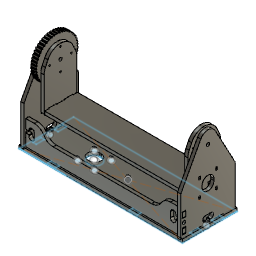
shotbot3 (Autodesk Fusion 360 design; units mm, degrees)
Autodesk Fusion 360 part; units mm, degrees
sketch "basetray sketch" plane through (0, 0, 0) normal (0, 0, 1) x (1, 0, 0) in component "Base Tray"
  line L0 (-147, -27.5) -> (-141, -27.5)
  line L1 (-85.5, -47) -> (-85.5, -41)
  arc A0 (-60.01, -11) -> (-60.01, 11) centre (-60.01, 0) ccw
  line L2 (-60.01, 11) -> (-63.01, 11)
  line L3 (-141, -27.5) -> (-141, -12.5)
  line L4 (-44.51, -14) -> (-47.51, -14)
  line L5 (147, 12.5) -> (147, 27.5)
  line L6 (-85.5, -41) -> (-100.5, -41)
  arc A1 (-78.51, -14) -> (-78.51, -17) centre (-78.51, -15.5) ccw
  line L7 (-100.5, -47) -> (-85.5, -47)
  line L8 (-100.5, -41) -> (-100.5, -47)
  line L9 (-147, 12.5) -> (-141, 12.5)
  line L10 (141, 27.5) -> (141, 12.5)
  arc A2 (-63.01, 11) -> (-63.01, -11) centre (-63.01, 0) ccw
  line L11 (-78.51, -17) -> (-75.51, -17)
  line L12 (-78.51, 14) -> (-75.51, 14)
  arc A3 (-47.51, -14) -> (-47.51, -17) centre (-47.51, -15.5) ccw
  line L13 (-150, 50) -> (150, 50)
  line L14 (-75.51, -14) -> (-78.51, -14)
  line L15 (49.5, -47) -> (64.5, -47)
  line L16 (150, 50) -> (150, -50)
  line L17 (141, 12.5) -> (147, 12.5)
  line L18 (147, -12.5) -> (141, -12.5)
  line L19 (64.5, -41) -> (49.5, -41)
  line L20 (-141, 27.5) -> (-147, 27.5)
  line L21 (-141, -12.5) -> (-147, -12.5)
  circle A4 centre (-144, 0) radius 3
  line L22 (-47.51, -17) -> (-44.51, -17)
  arc A5 (-44.51, -17) -> (-44.51, -14) centre (-44.51, -15.5) ccw
  line L23 (49.5, -41) -> (49.5, -47)
  arc A6 (-75.51, -17) -> (-75.51, -14) centre (-75.51, -15.5) ccw
  line L24 (-75.51, 17) -> (-78.51, 17)
  line L25 (-150, 50) -> (150, -50) construction
  line L26 (64.5, -47) -> (64.5, -41)
  arc A7 (-75.51, 14) -> (-75.51, 17) centre (-75.51, 15.5) ccw
  line L27 (-63.01, -11) -> (-60.01, -11)
  line L28 (-147, 27.5) -> (-147, 12.5)
  line L29 (141, -12.5) -> (141, -27.5)
  circle A8 centre (144, 0) radius 3
  arc A9 (-44.51, 14) -> (-44.51, 17) centre (-44.51, 15.5) ccw
  arc A10 (-47.51, 17) -> (-47.51, 14) centre (-47.51, 15.5) ccw
  line L30 (150, 50) -> (-150, -50) construction
  line L31 (150, -50) -> (-150, -50)
  line L32 (-147, -12.5) -> (-147, -27.5)
  arc A11 (-78.51, 17) -> (-78.51, 14) centre (-78.51, 15.5) ccw
  line L33 (141, -27.5) -> (147, -27.5)
  line L34 (147, -27.5) -> (147, -12.5)
  line L35 (-141, 12.5) -> (-141, 27.5)
  line L36 (-44.51, 17) -> (-47.51, 17)
  line L37 (-47.51, 14) -> (-44.51, 14)
  line L38 (147, 27.5) -> (141, 27.5)
  circle A12 centre (0, 0) radius 2.95
  line L39 (-150, -50) -> (-150, 50)
  constraint horizontal L13
  constraint perpendicular L13 L16
  constraint parallel L13 L31
  constraint parallel L16 L39
  constraint coincident A12.centre L25
  constraint coincident A12.centre L30
  constraint coincident A12.centre origin
sketch "Sketch1" plane through (0, 0, 0) normal (1, 0, 0) x (0, 1, 0) in component "Flange 2"
  line L0 (11, 69.99, -147) -> (11, 66.99, -147)
  arc A0 through (-5, 9, -147) (-10, 14, -147) (-5, 19, -147)
  line L1 (14, 51.49, -147) -> (14, 54.49, -147)
  line L2 (-47, 35.5, -147) -> (-47, 45.5, -147)
  arc A1 through (-17, 54.49, -147) (-15.5, 55.99, -147) (-14, 54.49, -147)
  line L3 (-3.2, 9, -147) -> (-5, 9, -147)
  line L4 (-47, 20.5, -147) -> (-41, 20.5, -147)
  arc A2 through (17, 82.49, -147) (15.5, 80.99, -147) (14, 82.49, -147)
  arc A3 through (5, 19, -147) (10, 14, -147) (5, 9, -147)
  arc A4 through (-17, 85.49, -147) (-15.5, 86.99, -147) (-14, 85.49, -147)
  line L5 (-47, 45.5, -147) -> (-41, 45.5, -147)
  arc A5 through (14, 85.49, -147) (15.5, 86.99, -147) (17, 85.49, -147)
  line L6 (-17, 82.49, -147) -> (-17, 85.49, -147)
  line L7 (17, 85.49, -147) -> (17, 82.49, -147)
  line L8 (-5, 19, -147) -> (5, 19, -147)
  circle A6 through (-2.9, 130, -147) (1.45, 132.5115, -147) (1.45, 127.4885, -147)
  line L9 (12.4, 3, -147) -> (3.2, 3, -147)
  line L10 (5, 9, -147) -> (3.2, 9, -147)
  line L11 (-3.2, 3, -147) -> (-3.2, 9, -147)
  line L12 (-27.3905, -3, -147) -> (-27.6, 3, -147)
  line L13 (-12.6095, -3, -147) -> (-27.3905, -3, -147)
  arc A7 through (14, 54.49, -147) (15.5, 55.99, -147) (17, 54.49, -147)
  line L14 (14, 82.49, -147) -> (14, 85.49, -147)
  arc A8 through (-11, 69.99, -147) (0, 80.99, -147) (11, 69.99, -147)
  line L15 (-41, 35.5, -147) -> (-47, 35.5, -147)
  line L16 (-41, 20.5, -147) -> (-41, 10.5, -147)
  line L17 (-12.4, 3, -147) -> (-12.6095, -3, -147)
  arc A9 through (17, 51.49, -147) (15.5, 49.99, -147) (14, 51.49, -147)
  circle A10 through (-47, 28, -147) (-42.5, 30.5981, -147) (-42.5, 25.4019, -147)
  line L18 (-17, 51.49, -147) -> (-17, 54.49, -147)
  line L19 (27.6, 3, -147) -> (27.3905, -3, -147)
  line L20 (-11, 66.99, -147) -> (-11, 69.99, -147)
  line L21 (-14, 85.49, -147) -> (-14, 82.49, -147)
  arc A11 through (-14, 51.49, -147) (-15.5, 49.99, -147) (-17, 51.49, -147)
  line L22 (27.3905, -3, -147) -> (12.6095, -3, -147)
  arc A12 through (-14, 82.49, -147) (-15.5, 80.99, -147) (-17, 82.49, -147)
  line L23 (-3.2, 3, -147) -> (-12.4, 3, -147)
  line L24 (-41, 45.5, -147) -> (-41, 35.5, -147)
  line L25 (-27.6, 3, -147) -> (-50, 3, -147)
  line L26 (-41, 10.5, -147) -> (-47, 10.5, -147)
  line L27 (12.6095, -3, -147) -> (12.4, 3, -147)
  line L28 (50, 76.6902, -147) -> (50, 3, -147)
  line L29 (-50, 3, -147) -> (-50, 76.6902, -147)
  line L30 (17, 54.49, -147) -> (17, 51.49, -147)
  line L31 (50, 3, -147) -> (27.6, 3, -147)
  line L32 (3.2, 9, -147) -> (3.2, 3, -147)
  arc A13 through (11, 66.99, -147) (0, 55.99, -147) (-11, 66.99, -147)
  line L33 (-47, 10.5, -147) -> (-47, 20.5, -147)
  line L34 (-14, 54.49, -147) -> (-14, 51.49, -147)
  line L35 (50, 76.6902, -147) -> (13.2596, 145.255, -147)
  line L36 (-13.2003, 145.2233, -147) -> (-50, 76.1506, -147)
  arc A14 through (13.2596, 145.255, -147) (0.0202, 153.1703, -147) (-13.2003, 145.2233, -147)
  dimension "d2" = 15
extrude "Extrude1" add sketch "Sketch1" along normal blind 6 contours A0 L3 A3 L8 L9 L10 L11 L12 L13 L17 L19 L22 L23 L25 L27 L28 L29 L31 L32 L35 L36 A14 in plane through (-147, 0, 0) normal (1, 0, 0) makes body 1 in component "Flange 2"
extrude "Extrude1'" add sketch "basetray sketch" along normal blind 6 separate body makes body 2 in component "Base Tray"
sketch "Sketch1 (2)" plane through (0, 0, 0) normal (0, 1, 0) x (1, 0, 0) in component "Back support"
  line L0 (-147, -20.1905, -49) -> (-141, -20.4, -49)
  line L1 (147, -45.1905, -49) -> (147, -35.9095, -49)
  arc A0 through (-125, -25.8, -49) (-130, -20.8, -49) (-135, -25.8, -49)
  line L2 (-135, -27.8, -49) -> (-135, -25.8, -49)
  line L3 (135, -25.8, -49) -> (135, -27.8, -49)
  line L4 (49.5, -5.8, -49) -> (-85.5, -5.8, -49)
  line L5 (49.7095, 0.2, -49) -> (49.5, -5.8, -49)
  arc A1 through (125, -35.8, -49) (130, -40.8, -49) (135, -35.8, -49)
  line L6 (-141, -45.4, -49) -> (-141, -50.8, -49)
  line L7 (125, -35.8, -49) -> (125, -25.8, -49)
  line L8 (-141, -20.4, -49) -> (-141, -27.8, -49)
  line L9 (64.5, -5.8, -49) -> (64.2905, 0.2, -49)
  line L10 (-141, -5.8, -49) -> (-141, -10.6, -49)
  line L11 (141, -27.8, -49) -> (141, -18.9, -49)
  arc A2 through (-90.359, -30.8, -49) (-100.359, -33.4795, -49) (-107.6795, -40.8, -49)
  line L12 (64.2905, 0.2, -49) -> (49.7095, 0.2, -49)
  line L13 (125, -50.8, -49) -> (141, -50.8, -49)
  line L14 (147, -18.6905, -49) -> (147, -9.3095, -49)
  line L15 (-135, -33.8, -49) -> (-141, -33.8, -49)
  arc A3 through (-125, -50.8, -49) (-115, -48.1205, -49) (-107.6795, -40.8, -49)
  line L16 (-85.7095, 0.2, -49) -> (-100.2905, 0.2, -49)
  line L17 (-141, -27.8, -49) -> (-135, -27.8, -49)
  line L18 (-141, -50.8, -49) -> (-125, -50.8, -49)
  line L19 (141, -5.8, -49) -> (64.5, -5.8, -49)
  line L20 (141, -9.1, -49) -> (141, -5.8, -49)
  line L21 (-90.359, -30.8, -49) -> (90.359, -30.8, -49)
  line L22 (-135, -35.8, -49) -> (-135, -33.8, -49)
  arc A4 through (107.6795, -40.8, -49) (115, -48.1205, -49) (125, -50.8, -49)
  line L23 (-100.5, -5.8, -49) -> (-141, -5.8, -49)
  arc A5 through (107.6795, -40.8, -49) (100.359, -33.4795, -49) (90.359, -30.8, -49)
  line L24 (135, -33.8, -49) -> (135, -35.8, -49)
  line L25 (135, -27.8, -49) -> (141, -27.8, -49)
  arc A6 through (135, -25.8, -49) (130, -20.8, -49) (125, -25.8, -49)
  line L26 (-100.2905, 0.2, -49) -> (-100.5, -5.8, -49)
  line L27 (141, -18.9, -49) -> (147, -18.6905, -49)
  line L28 (-125, -25.8, -49) -> (-125, -35.8, -49)
  line L29 (-147, -10.8095, -49) -> (-147, -20.1905, -49)
  arc A7 through (-135, -35.8, -49) (-130, -40.8, -49) (-125, -35.8, -49)
  line L30 (-85.5, -5.8, -49) -> (-85.7095, 0.2, -49)
  line L31 (141, -33.8, -49) -> (135, -33.8, -49)
  line L32 (-141, -10.6, -49) -> (-147, -10.8095, -49)
  line L33 (-141, -33.8, -49) -> (-141, -35.7, -49)
  line L34 (141, -35.7, -49) -> (141, -33.8, -49)
  line L35 (-147, -35.9095, -49) -> (-147, -45.1905, -49)
  line L36 (141, -45.4, -49) -> (147, -45.1905, -49)
  line L37 (147, -9.3095, -49) -> (141, -9.1, -49)
  line L38 (141, -50.8, -49) -> (141, -45.4, -49)
  line L39 (-147, -45.1905, -49) -> (-141, -45.4, -49)
  line L40 (-141, -35.7, -49) -> (-147, -35.9095, -49)
  line L41 (147, -35.9095, -49) -> (141, -35.7, -49)
extrude "Extrude1''" add sketch "Sketch1 (2)" along normal blind 6 separate body contours L0 L1 A0 L2 L3 L4 L5 A1 L6 L7 L8 L9 L10 L11 A2 L12 L13 L14 L15 A3 L16 L17 L18 L19 L20 L21 L22 A4 L23 A5 L24 L25 A6 L26 L27 L28 L29 A7 L30 L31 L32 L33 L34 L35 L36 L37 L38 L39 L40 L41 in plane through (0, -49, 0) normal (0, 1, 0) makes body 3 in component "Back support"
sketch "Sketch1 (3)" plane through (-147, 0, 0) normal (-1, 0, 0) x (0, -1, 0) in component "Tilt Flange 2"
  line L0 (-11, 66.99) -> (-11, 69.99)
  arc A0 (11, 69.99) -> (-11, 69.99) centre (0, 69.99) ccw
  line L1 (11, 69.99) -> (11, 66.99)
  arc A1 (-11, 66.99) -> (11, 66.99) centre (0, 66.99) ccw
  arc A2 (-14, 54.49) -> (-17, 54.49) centre (-15.5, 54.49) ccw
  line L2 (-14, 54.49) -> (-14, 51.49)
  arc A3 (-17, 51.49) -> (-14, 51.49) centre (-15.5, 51.49) ccw
  line L3 (-17, 51.49) -> (-17, 54.49)
  line L4 (14, 82.49) -> (14, 85.49)
  arc A4 (17, 85.49) -> (14, 85.49) centre (15.5, 85.49) ccw
  line L5 (17, 85.49) -> (17, 82.49)
  arc A5 (14, 82.49) -> (17, 82.49) centre (15.5, 82.49) ccw
  line L6 (47, 10.5) -> (41, 10.5)
  line L7 (41, 10.5) -> (41, 20.5)
  line L8 (41, 20.5) -> (47, 20.5)
  line L9 (47, 20.5) -> (47, 10.5)
  circle A6 centre (44, 28) radius 3
  arc A7 (17, 54.49) -> (14, 54.49) centre (15.5, 54.49) ccw
  line L10 (17, 54.49) -> (17, 51.49)
  arc A8 (14, 51.49) -> (17, 51.49) centre (15.5, 51.49) ccw
  line L11 (14, 51.49) -> (14, 54.49)
  circle A9 centre (0, 130) radius 2.9
  line L12 (41, 45.5) -> (47, 45.5)
  line L13 (47, 45.5) -> (47, 35.5)
  line L14 (47, 35.5) -> (41, 35.5)
  line L15 (41, 35.5) -> (41, 45.5)
  arc A10 (-17, 82.49) -> (-14, 82.49) centre (-15.5, 82.49) ccw
  line L16 (-17, 82.49) -> (-17, 85.49)
  arc A11 (-14, 85.49) -> (-17, 85.49) centre (-15.5, 85.49) ccw
  line L17 (-14, 85.49) -> (-14, 82.49)
  line L18 (-13.2596, 145.255) -> (-50, 76.6902)
  line L19 (-50, 76.6902) -> (-50, 3)
  line L20 (-50, 3) -> (-27.6, 3)
  line L21 (-27.6, 3) -> (-27.3905, -3)
  line L22 (-27.3905, -3) -> (-12.6095, -3)
  line L23 (-12.6095, -3) -> (-12.4, 3)
  line L24 (-12.4, 3) -> (-3.2, 3)
  line L25 (-3.2, 3) -> (-3.2, 9)
  line L26 (-3.2, 9) -> (-5, 9)
  arc A12 (-5, 19) -> (-5, 9) centre (-5, 14) ccw
  line L27 (-5, 19) -> (5, 19)
  arc A13 (5, 9) -> (5, 19) centre (5, 14) ccw
  line L28 (5, 9) -> (3.2, 9)
  line L29 (3.2, 9) -> (3.2, 3)
  line L30 (3.2, 3) -> (12.4, 3)
  line L31 (12.4, 3) -> (12.6095, -3)
  line L32 (12.6095, -3) -> (27.3905, -3)
  line L33 (27.3905, -3) -> (27.6, 3)
  line L34 (27.6, 3) -> (50, 3)
  line L35 (50, 3) -> (50, 76.1506)
  line L36 (50, 76.1506) -> (13.2003, 145.2233)
  arc A14 (13.2003, 145.2233) -> (-13.2596, 145.255) centre (-0.0381, 138.1703) ccw
  line L37 (-7.5, 63, -8) -> (-22.5, 63, -8)
  line L38 (-23.0202, 140.7345, -8) -> (-27.6202, 130.8698, -8)
  line L39 (22.5, 63, -8) -> (7.5, 63, -8)
  line L40 (-22.5, 57, -8) -> (-7.5, 57, -8)
  line L41 (7.5, 57, -8) -> (22.5, 57, -8)
  line L42 (30, 57.8416, -8) -> (30, 120.1353, -8)
  line L43 (-30, 120.1353, -8) -> (-30, 57.4169, -8)
  circle A15 through (21.5, 130, -8) (19.25, 131.299, -8) (19.25, 128.701, -8)
  arc A16 through (23.0202, 140.7345, -8) (0, 155.4, -8) (-23.0202, 140.7345, -8)
  line L44 (27.6202, 130.8698, -8) -> (23.0202, 140.7345, -8)
  arc A17 through (23.9043, 54.4345, -8) (27.9516, 54.35, -8) (30, 57.8416, -8)
  line L45 (22.5, 57, -8) -> (22.5, 63, -8)
  line L46 (-22.5, 63, -8) -> (-22.5, 57, -8)
  arc A18 through (30, 120.1353, -8) (29.3979, 125.6328, -8) (27.6202, 130.8698, -8)
  circle A19 through (1.5, 150, -8) (-0.75, 151.299, -8) (-0.75, 148.701, -8)
  circle A20 through (2.95, 130, -8) (-1.475, 132.5548, -8) (-1.475, 127.4452, -8)
  arc A21 through (-30, 57.4169, -8) (-27.7787, 54.2343, -8) (-23.9027, 54.4345, -8)
  line L47 (-23.9027, 54.4345, -8) -> (23.9043, 54.4345, -8)
  arc A22 through (-27.6202, 130.8698, -8) (-29.3979, 125.6328, -8) (-30, 120.1353, -8)
  line L48 (7.5, 63, -8) -> (7.5, 57, -8)
  circle A23 through (1.5, 110, -8) (-0.75, 111.299, -8) (-0.75, 108.701, -8)
  line L49 (-7.5, 57, -8) -> (-7.5, 63, -8)
  circle A24 through (-18.5, 130, -8) (-20.75, 131.299, -8) (-20.75, 128.701, -8)
  point P0 (0, 130)
extrude "Extrude1'''" add sketch "Sketch1 (3)" against normal blind 6 separate body contours L38 L42 L43 A16 L44 A17 A18 A21 L47 A22 in plane through (-139, 0, 0) normal (-1, 0, 0) makes body 4 in component "Tilt Flange 2"
sketch "Sketch1 (4)" plane through (0, 0, 0) normal (1, 0, 0) x (0, 1, 0) in component "Large gear"
  line L0 (-18.2151, 96.9927, -130) -> (-18.3358, 95.6128, -130)
  line L1 (36.8786, 133.8051, -130) -> (38.1997, 133.3886, -130)
  arc A0 through (34.008, 144.5186, -130) (33.9137, 144.3273, -130) (33.9369, 144.1154, -130)
  line L2 (-15.0693, 95.4413, -130) -> (-16.0905, 94.5056, -130)
  arc A1 through (3.5993, 167.9889, -130) (2.3516, 168.0911, -130) (1.1012, 168.1527, -130)
  arc A2 through (-4.6694, 166.4048, -130) (-4.4743, 166.4906, -130) (-4.3558, 166.6679, -130)
  line L3 (-0.5105, 166.6774, -130) -> (0.1705, 166.6774, -130)
  line L4 (-10.4807, 165.4496, -130) -> (-11.371, 166.5107, -130)
  line L5 (-32.1108, 148.8522, -130) -> (-32.9053, 149.9869, -130)
  line L6 (-36.9554, 134.1188, -130) -> (-36.8666, 134.7939, -130)
  line L7 (-34.5375, 143.4862, -130) -> (-34.2769, 144.1154, -130)
  line L8 (-32.4334, 147.8535, -130) -> (-32.0929, 148.4432, -130)
  arc A3 through (-36.8666, 134.7939, -130) (-36.899, 135.0047, -130) (-37.0396, 135.165, -130)
  arc A4 through (-35.8772, 139.5395, -130) (-35.8818, 139.7527, -130) (-36.0003, 139.93, -130)
  line L9 (-37.0396, 135.165, -130) -> (-38.2078, 135.9092, -130)
  line L10 (-34.8728, 143.2514, -130) -> (-36.2566, 143.191, -130)
  line L11 (-37.2186, 133.8051, -130) -> (-38.5396, 133.3886, -130)
  line L12 (-37.448, 130.3051, -130) -> (-38.7034, 130.8905, -130)
  line L13 (-36.0534, 138.8817, -130) -> (-35.8772, 139.5395, -130)
  arc A5 through (-37.448, 128.9335, -130) (-37.2877, 129.0741, -130) (-37.228, 129.2788, -130)
  arc A6 through (-38.5396, 133.3886, -130) (-38.6418, 132.1409, -130) (-38.7034, 130.8905, -130)
  arc A7 through (-34.1765, 147.7851, -130) (-34.7483, 146.6715, -130) (-35.2837, 145.5398, -130)
  arc A8 through (-34.8728, 143.2514, -130) (-34.6709, 143.3199, -130) (-34.5375, 143.4862, -130)
  arc A9 through (-37.228, 129.9598, -130) (-37.2877, 130.1645, -130) (-37.448, 130.3051, -130)
  arc A10 through (-32.0929, 148.4432, -130) (-32.0423, 148.6503, -130) (-32.1108, 148.8522, -130)
  arc A11 through (-37.7194, 138.3646, -130) (-37.9835, 137.1409, -130) (-38.2078, 135.9092, -130)
  line L14 (-32.7966, 147.6644, -130) -> (-34.1765, 147.7851, -130)
  line L15 (-36.0003, 139.93, -130) -> (-37.0614, 140.8203, -130)
  arc A12 through (-36.3553, 138.6051, -130) (-36.1641, 138.6994, -130) (-36.0534, 138.8817, -130)
  arc A13 through (-37.2186, 133.8051, -130) (-37.0413, 133.9236, -130) (-36.9554, 134.1188, -130)
  arc A14 through (-32.7966, 147.6644, -130) (-32.5875, 147.706, -130) (-32.4334, 147.8535, -130)
  arc A15 through (-34.2769, 144.1154, -130) (-34.2536, 144.3273, -130) (-34.3479, 144.5186, -130)
  circle A16 through (-19.42, 129.6193, -130) (-20.545, 130.2688, -130) (-20.545, 128.9698, -130)
  line L16 (-37.228, 129.2788, -130) -> (-37.228, 129.9598, -130)
  line L17 (-36.3553, 138.6051, -130) -> (-37.7194, 138.3646, -130)
  line L18 (-37.448, 128.9335, -130) -> (-38.7034, 128.3481, -130)
  line L19 (-34.3479, 144.5186, -130) -> (-35.2837, 145.5398, -130)
  arc A17 through (-36.2566, 143.191, -130) (-36.6782, 142.0122, -130) (-37.0614, 140.8203, -130)
  line L20 (-14.6661, 163.7262, -130) -> (-14.0369, 163.9868, -130)
  line L21 (-26.6147, 155.5825, -130) -> (-26.1332, 156.0641, -130)
  line L22 (-23.4075, 158.7765, -130) -> (-24.6361, 159.416, -130)
  line L23 (-30.1621, 151.7687, -130) -> (-31.5144, 152.0684, -130)
  line L24 (-15.0693, 163.7973, -130) -> (-16.0905, 164.733, -130)
  arc A18 through (-27.0145, 155.4939, -130) (-26.8017, 155.48, -130) (-26.6147, 155.5825, -130)
  arc A19 through (-24.6361, 159.416, -130) (-25.5906, 158.606, -130) (-26.5183, 157.7654, -130)
  arc A20 through (-19.4029, 161.5601, -130) (-19.201, 161.4916, -130) (-18.9939, 161.5423, -130)
  arc A21 through (-28.3161, 155.9677, -130) (-29.1567, 155.0399, -130) (-29.9667, 154.0854, -130)
  arc A22 through (-23.4075, 158.7765, -130) (-23.1984, 158.7349, -130) (-22.9996, 158.8122, -130)
  arc A23 through (-14.0369, 163.9868, -130) (-13.8706, 164.1202, -130) (-13.8021, 164.3222, -130)
  line L25 (-18.9939, 161.5423, -130) -> (-18.4041, 161.8828, -130)
  line L26 (-29.7774, 151.9087, -130) -> (-29.3628, 152.449, -130)
  arc A24 through (-18.4041, 161.8828, -130) (-18.2567, 162.0368, -130) (-18.2151, 162.2459, -130)
  arc A25 through (-26.1332, 156.0641, -130) (-26.0307, 156.251, -130) (-26.0446, 156.4638, -130)
  arc A26 through (-30.1621, 151.7687, -130) (-29.9493, 151.7826, -130) (-29.7774, 151.9087, -130)
  line L27 (-22.3193, 159.6114, -130) -> (-22.6191, 160.9637, -130)
  line L28 (-19.4029, 161.5601, -130) -> (-20.5375, 162.3546, -130)
  line L29 (-26.0446, 156.4638, -130) -> (-26.5183, 157.7654, -130)
  line L30 (-29.3271, 152.8568, -130) -> (-29.9667, 154.0854, -130)
  line L31 (-13.8021, 164.3222, -130) -> (-13.7417, 165.706, -130)
  arc A27 through (-22.4594, 159.2267, -130) (-22.3333, 159.3987, -130) (-22.3193, 159.6114, -130)
  arc A28 through (-29.3628, 152.449, -130) (-29.2855, 152.6477, -130) (-29.3271, 152.8568, -130)
  arc A29 through (-16.0905, 164.733, -130) (-17.2221, 164.1976, -130) (-18.3358, 163.6258, -130)
  arc A30 through (-15.0693, 163.7973, -130) (-14.878, 163.703, -130) (-14.6661, 163.7262, -130)
  arc A31 through (-31.5144, 152.0684, -130) (-32.2267, 151.0389, -130) (-32.9053, 149.9869, -130)
  arc A32 through (-20.5375, 162.3546, -130) (-21.5896, 161.6761, -130) (-22.6191, 160.9637, -130)
  line L32 (-27.0145, 155.4939, -130) -> (-28.3161, 155.9677, -130)
  line L33 (-18.2151, 162.2459, -130) -> (-18.3358, 163.6258, -130)
  line L34 (-22.9996, 158.8122, -130) -> (-22.4594, 159.2267, -130)
  arc A33 through (-11.371, 166.5107, -130) (-12.5629, 166.1276, -130) (-13.7417, 165.706, -130)
  line L35 (-29.3271, 106.3818, -130) -> (-29.9667, 105.1532, -130)
  line L36 (-30.1621, 107.47, -130) -> (-31.5144, 107.1702, -130)
  line L37 (-26.0446, 102.7748, -130) -> (-26.5183, 101.4732, -130)
  arc A34 through (-18.3358, 95.6128, -130) (-17.2221, 95.041, -130) (-16.0905, 94.5056, -130)
  line L38 (36.0153, 138.6051, -130) -> (37.3794, 138.3646, -130)
  arc A35 through (-22.9996, 100.4265, -130) (-23.1984, 100.5037, -130) (-23.4075, 100.4621, -130)
  line L39 (25.7046, 156.4638, -130) -> (26.1784, 157.7654, -130)
  arc A36 through (29.6268, 154.0854, -130) (28.8167, 155.0399, -130) (27.9761, 155.9677, -130)
  arc A37 through (-32.4334, 111.3852, -130) (-32.5875, 111.5326, -130) (-32.7966, 111.5742, -130)
  line L40 (-36.0003, 119.3086, -130) -> (-37.0614, 118.4183, -130)
  line L41 (-34.8728, 115.9872, -130) -> (-36.2566, 116.0476, -130)
  arc A38 through (-34.3479, 114.72, -130) (-34.2536, 114.9113, -130) (-34.2769, 115.1232, -130)
  arc A39 through (22.2792, 160.9637, -130) (21.2497, 161.6761, -130) (20.1976, 162.3546, -130)
  arc A40 through (29.4374, 151.9087, -130) (29.6094, 151.7826, -130) (29.8222, 151.7687, -130)
  arc A41 through (-37.0614, 118.4183, -130) (-36.6782, 117.2264, -130) (-36.2566, 116.0476, -130)
  line L42 (26.6745, 155.4939, -130) -> (27.9761, 155.9677, -130)
  arc A42 through (26.2748, 155.5825, -130) (26.4617, 155.48, -130) (26.6745, 155.4939, -130)
  line L43 (29.8222, 151.7687, -130) -> (31.1744, 152.0684, -130)
  line L44 (25.7932, 156.0641, -130) -> (26.2748, 155.5825, -130)
  line L45 (22.1194, 159.2267, -130) -> (22.6597, 158.8122, -130)
  arc A43 through (22.6597, 158.8122, -130) (22.8584, 158.7349, -130) (23.0675, 158.7765, -130)
  arc A44 through (-36.9554, 125.1198, -130) (-37.0413, 125.315, -130) (-37.2186, 125.4335, -130)
  line L46 (-32.7966, 111.5742, -130) -> (-34.1765, 111.4535, -130)
  line L47 (21.9794, 159.6114, -130) -> (22.2792, 160.9637, -130)
  line L48 (33.9369, 144.1154, -130) -> (34.1975, 143.4862, -130)
  arc A45 through (34.1975, 143.4862, -130) (34.331, 143.3199, -130) (34.5329, 143.2514, -130)
  arc A46 through (31.7708, 148.8522, -130) (31.7023, 148.6503, -130) (31.753, 148.4432, -130)
  arc A47 through (35.7135, 138.8817, -130) (35.8241, 138.6994, -130) (36.0153, 138.6051, -130)
  arc A48 through (36.6155, 134.1188, -130) (36.7014, 133.9236, -130) (36.8786, 133.8051, -130)
  line L49 (23.0675, 158.7765, -130) -> (24.2961, 159.416, -130)
  line L50 (-36.8666, 124.4447, -130) -> (-36.9554, 125.1198, -130)
  line L51 (29.0229, 152.449, -130) -> (29.4374, 151.9087, -130)
  line L52 (-34.2769, 115.1232, -130) -> (-34.5375, 115.7524, -130)
  arc A49 through (21.9794, 159.6114, -130) (21.9933, 159.3987, -130) (22.1194, 159.2267, -130)
  arc A50 through (35.6603, 139.93, -130) (35.5419, 139.7527, -130) (35.5372, 139.5395, -130)
  line L53 (-18.4041, 97.3558, -130) -> (-18.9939, 97.6963, -130)
  arc A51 through (37.8678, 135.9092, -130) (37.6435, 137.1409, -130) (37.3794, 138.3646, -130)
  line L54 (31.753, 148.4432, -130) -> (32.0935, 147.8535, -130)
  arc A52 through (-29.9667, 105.1532, -130) (-29.1567, 104.1987, -130) (-28.3161, 103.2709, -130)
  line L55 (34.5329, 143.2514, -130) -> (35.9167, 143.191, -130)
  line L56 (36.5266, 134.7939, -130) -> (36.6155, 134.1188, -130)
  arc A53 through (32.5653, 149.9869, -130) (31.8868, 151.0389, -130) (31.1744, 152.0684, -130)
  arc A54 through (-26.5183, 101.4732, -130) (-25.5906, 100.6326, -130) (-24.6361, 99.8226, -130)
  line L57 (34.008, 144.5186, -130) -> (34.9438, 145.5398, -130)
  arc A55 through (-29.3271, 106.3818, -130) (-29.2855, 106.5909, -130) (-29.3628, 106.7897, -130)
  arc A56 through (36.7214, 140.8203, -130) (36.3383, 142.0122, -130) (35.9167, 143.191, -130)
  arc A57 through (32.0935, 147.8535, -130) (32.2475, 147.706, -130) (32.4566, 147.6644, -130)
  arc A58 through (-18.2151, 96.9927, -130) (-18.2567, 97.2018, -130) (-18.4041, 97.3558, -130)
  arc A59 through (36.6996, 135.165, -130) (36.559, 135.0047, -130) (36.5266, 134.7939, -130)
  arc A60 through (-22.3193, 99.6272, -130) (-22.3333, 99.8399, -130) (-22.4594, 100.0119, -130)
  line L58 (35.5372, 139.5395, -130) -> (35.7135, 138.8817, -130)
  line L59 (35.6603, 139.93, -130) -> (36.7214, 140.8203, -130)
  arc A61 through (-14.6661, 95.5124, -130) (-14.878, 95.5356, -130) (-15.0693, 95.4413, -130)
  arc A62 through (-26.0446, 102.7748, -130) (-26.0307, 102.9876, -130) (-26.1332, 103.1745, -130)
  arc A63 through (34.9438, 145.5398, -130) (34.4084, 146.6715, -130) (33.8365, 147.7851, -130)
  arc A64 through (-37.0396, 124.0736, -130) (-36.899, 124.2339, -130) (-36.8666, 124.4447, -130)
  arc A65 through (28.9872, 152.8568, -130) (28.9456, 152.6477, -130) (29.0229, 152.449, -130)
  arc A66 through (-32.1108, 110.3864, -130) (-32.0423, 110.5883, -130) (-32.0929, 110.7954, -130)
  arc A67 through (26.1784, 157.7654, -130) (25.2507, 158.606, -130) (24.2961, 159.416, -130)
  arc A68 through (25.7046, 156.4638, -130) (25.6907, 156.251, -130) (25.7932, 156.0641, -130)
  line L60 (-37.2186, 125.4335, -130) -> (-38.5396, 125.85, -130)
  line L61 (28.9872, 152.8568, -130) -> (29.6268, 154.0854, -130)
  line L62 (-32.0929, 110.7954, -130) -> (-32.4334, 111.3852, -130)
  arc A69 through (-38.7034, 128.3481, -130) (-38.6418, 127.0977, -130) (-38.5396, 125.85, -130)
  arc A70 through (-35.2837, 113.6988, -130) (-34.7483, 112.5672, -130) (-34.1765, 111.4535, -130)
  arc A71 through (-34.5375, 115.7524, -130) (-34.6709, 115.9187, -130) (-34.8728, 115.9872, -130)
  arc A72 through (-36.0003, 119.3086, -130) (-35.8818, 119.4859, -130) (-35.8772, 119.6991, -130)
  line L63 (-32.1108, 110.3864, -130) -> (-32.9053, 109.2517, -130)
  line L64 (-35.8772, 119.6991, -130) -> (-36.0534, 120.3569, -130)
  line L65 (-37.0396, 124.0736, -130) -> (-38.2078, 123.3294, -130)
  line L66 (-36.3553, 120.6335, -130) -> (-37.7194, 120.874, -130)
  line L67 (-34.3479, 114.72, -130) -> (-35.2837, 113.6988, -130)
  arc A73 through (-38.2078, 123.3294, -130) (-37.9835, 122.0977, -130) (-37.7194, 120.874, -130)
  arc A74 through (-36.0534, 120.3569, -130) (-36.1641, 120.5392, -130) (-36.3553, 120.6335, -130)
  circle A75 through (2.83, 129.6193, -130) (-1.67, 132.2174, -130) (-1.67, 127.0212, -130)
  circle A76 through (20.58, 129.6193, -130) (19.455, 130.2688, -130) (19.455, 128.9698, -130)
  circle A77 through (2.83, 129.6193, -130) (-1.67, 132.2174, -130) (-1.67, 127.0212, -130)
  circle A78 through (0.58, 149.6193, -130) (-0.545, 150.2688, -130) (-0.545, 148.9698, -130)
  arc A79 through (13.4621, 164.3222, -130) (13.5306, 164.1202, -130) (13.6969, 163.9868, -130)
  arc A80 through (17.8751, 162.2459, -130) (17.9167, 162.0368, -130) (18.0642, 161.8828, -130)
  arc A81 through (5.0046, 166.3159, -130) (5.2154, 166.3483, -130) (5.3757, 166.4889, -130)
  line L68 (13.4621, 164.3222, -130) -> (13.4017, 165.706, -130)
  line L69 (19.063, 161.5601, -130) -> (20.1976, 162.3546, -130)
  line L70 (8.8159, 165.8046, -130) -> (8.5753, 167.1687, -130)
  line L71 (18.0642, 161.8828, -130) -> (18.6539, 161.5423, -130)
  arc A82 through (9.7502, 165.3265, -130) (9.9634, 165.3312, -130) (10.1407, 165.4496, -130)
  line L72 (9.0925, 165.5028, -130) -> (9.7502, 165.3265, -130)
  line L73 (13.6969, 163.9868, -130) -> (14.3261, 163.7262, -130)
  line L74 (4.0158, 166.6679, -130) -> (3.5993, 167.9889, -130)
  arc A83 through (17.9958, 163.6258, -130) (16.8822, 164.1976, -130) (15.7505, 164.733, -130)
  line L75 (14.7293, 163.7973, -130) -> (15.7505, 164.733, -130)
  line L76 (5.3757, 166.4889, -130) -> (6.1199, 167.6571, -130)
  line L77 (10.1407, 165.4496, -130) -> (11.0311, 166.5107, -130)
  arc A84 through (13.4017, 165.706, -130) (12.2229, 166.1276, -130) (11.0311, 166.5107, -130)
  arc A85 through (14.3261, 163.7262, -130) (14.5381, 163.703, -130) (14.7293, 163.7973, -130)
  arc A86 through (18.6539, 161.5423, -130) (18.861, 161.4916, -130) (19.063, 161.5601, -130)
  arc A87 through (8.5753, 167.1687, -130) (7.3516, 167.4328, -130) (6.1199, 167.6571, -130)
  arc A88 through (8.8159, 165.8046, -130) (8.9102, 165.6134, -130) (9.0925, 165.5028, -130)
  arc A89 through (4.0158, 166.6679, -130) (4.1343, 166.4906, -130) (4.3295, 166.4048, -130)
  line L78 (4.3295, 166.4048, -130) -> (5.0046, 166.3159, -130)
  line L79 (17.8751, 162.2459, -130) -> (17.9958, 163.6258, -130)
  arc A90 through (-0.8558, 166.8973, -130) (-0.7152, 166.737, -130) (-0.5105, 166.6774, -130)
  arc A91 through (-6.4599, 167.6571, -130) (-7.6916, 167.4328, -130) (-8.9153, 167.1687, -130)
  line L80 (-10.0902, 165.3265, -130) -> (-9.4324, 165.5028, -130)
  line L81 (-5.7157, 166.4889, -130) -> (-6.4599, 167.6571, -130)
  line L82 (-5.3446, 166.3159, -130) -> (-4.6694, 166.4048, -130)
  arc A92 through (0.1705, 166.6774, -130) (0.3752, 166.737, -130) (0.5158, 166.8973, -130)
  arc A93 through (-5.7157, 166.4889, -130) (-5.5554, 166.3483, -130) (-5.3446, 166.3159, -130)
  line L83 (-9.1558, 165.8046, -130) -> (-8.9153, 167.1687, -130)
  arc A94 through (-9.4324, 165.5028, -130) (-9.2501, 165.6134, -130) (-9.1558, 165.8046, -130)
  arc A95 through (-1.4412, 168.1527, -130) (-2.6916, 168.0911, -130) (-3.9393, 167.9889, -130)
  line L84 (0.5158, 166.8973, -130) -> (1.1012, 168.1527, -130)
  line L85 (-4.3558, 166.6679, -130) -> (-3.9393, 167.9889, -130)
  line L86 (-0.8558, 166.8973, -130) -> (-1.4412, 168.1527, -130)
  arc A96 through (-10.4807, 165.4496, -130) (-10.3034, 165.3312, -130) (-10.0902, 165.3265, -130)
  line L87 (36.6996, 135.165, -130) -> (37.8678, 135.9092, -130)
  arc A97 through (-18.9939, 97.6963, -130) (-19.201, 97.747, -130) (-19.4029, 97.6785, -130)
  line L88 (21.9794, 99.6272, -130) -> (22.2792, 98.2749, -130)
  line L89 (14.7293, 95.4413, -130) -> (15.7505, 94.5056, -130)
  arc A98 through (14.7293, 95.4413, -130) (14.5381, 95.5356, -130) (14.3261, 95.5124, -130)
  arc A99 through (23.0675, 100.4621, -130) (22.8584, 100.5037, -130) (22.6597, 100.4265, -130)
  line L90 (4.0158, 92.5707, -130) -> (3.5993, 91.2497, -130)
  arc A100 through (4.3295, 92.8338, -130) (4.1343, 92.748, -130) (4.0158, 92.5707, -130)
  arc A101 through (25.7932, 103.1745, -130) (25.6907, 102.9876, -130) (25.7046, 102.7748, -130)
  arc A102 through (9.0925, 93.7358, -130) (8.9102, 93.6252, -130) (8.8159, 93.434, -130)
  arc A103 through (26.6745, 103.7447, -130) (26.4617, 103.7586, -130) (26.2748, 103.6561, -130)
  line L91 (0.5158, 92.3413, -130) -> (1.1012, 91.0859, -130)
  line L92 (-4.3558, 92.5707, -130) -> (-3.9393, 91.2497, -130)
  line L93 (9.7502, 93.9121, -130) -> (9.0925, 93.7358, -130)
  line L94 (-5.7157, 92.7497, -130) -> (-6.4599, 91.5815, -130)
  line L95 (0.1705, 92.5613, -130) -> (-0.5105, 92.5613, -130)
  line L96 (36.8881, 129.9598, -130) -> (36.8881, 129.2788, -130)
  line L97 (22.6597, 100.4265, -130) -> (22.1194, 100.0119, -130)
  line L98 (-10.4807, 93.789, -130) -> (-11.371, 92.7279, -130)
  arc A104 through (-3.9393, 91.2497, -130) (-2.6916, 91.1475, -130) (-1.4412, 91.0859, -130)
  line L99 (18.6539, 97.6963, -130) -> (18.0642, 97.3558, -130)
  line L100 (36.8786, 125.4335, -130) -> (38.1997, 125.85, -130)
  arc A105 through (-9.1558, 93.434, -130) (-9.2501, 93.6252, -130) (-9.4324, 93.7358, -130)
  arc A106 through (-0.5105, 92.5613, -130) (-0.7152, 92.5016, -130) (-0.8558, 92.3413, -130)
  arc A107 through (33.8365, 111.4535, -130) (34.4084, 112.5672, -130) (34.9438, 113.6988, -130)
  line L101 (34.1975, 115.7524, -130) -> (33.9369, 115.1232, -130)
  line L102 (-0.8558, 92.3413, -130) -> (-1.4412, 91.0859, -130)
  line L103 (-9.1558, 93.434, -130) -> (-8.9153, 92.0699, -130)
  line L104 (37.1081, 128.9335, -130) -> (38.3634, 128.3481, -130)
  arc A108 through (10.1407, 93.789, -130) (9.9634, 93.9075, -130) (9.7502, 93.9121, -130)
  arc A109 through (0.5158, 92.3413, -130) (0.3752, 92.5016, -130) (0.1705, 92.5613, -130)
  arc A110 through (29.8222, 107.47, -130) (29.6094, 107.456, -130) (29.4374, 107.3299, -130)
  line L105 (36.0153, 120.6335, -130) -> (37.3794, 120.874, -130)
  arc A111 through (5.3757, 92.7497, -130) (5.2154, 92.8903, -130) (5.0046, 92.9227, -130)
  circle A112 through (0.58, 109.6193, -130) (-0.545, 110.2688, -130) (-0.545, 108.9698, -130)
  arc A113 through (35.5372, 119.6991, -130) (35.5419, 119.4859, -130) (35.6603, 119.3086, -130)
  line L106 (14.3261, 95.5124, -130) -> (13.6969, 95.2518, -130)
  arc A114 through (-5.3446, 92.9227, -130) (-5.5554, 92.8903, -130) (-5.7157, 92.7497, -130)
  arc A115 through (32.4566, 111.5742, -130) (32.2475, 111.5326, -130) (32.0935, 111.3852, -130)
  line L107 (-4.6694, 92.8338, -130) -> (-5.3446, 92.9227, -130)
  line L108 (-9.4324, 93.7358, -130) -> (-10.0902, 93.9121, -130)
  line L109 (29.8222, 107.47, -130) -> (31.1744, 107.1702, -130)
  arc A116 through (33.9369, 115.1232, -130) (33.9137, 114.9113, -130) (34.008, 114.72, -130)
  arc A117 through (-10.0902, 93.9121, -130) (-10.3034, 93.9075, -130) (-10.4807, 93.789, -130)
  arc A118 through (20.1976, 96.884, -130) (21.2497, 97.5625, -130) (22.2792, 98.2749, -130)
  line L110 (5.3757, 92.7497, -130) -> (6.1199, 91.5815, -130)
  arc A119 through (37.3794, 120.874, -130) (37.6435, 122.0977, -130) (37.8678, 123.3294, -130)
  arc A120 through (-4.3558, 92.5707, -130) (-4.4743, 92.748, -130) (-4.6694, 92.8338, -130)
  arc A121 through (36.0153, 120.6335, -130) (35.8241, 120.5392, -130) (35.7135, 120.3569, -130)
  arc A122 through (1.1012, 91.0859, -130) (2.3516, 91.1475, -130) (3.5993, 91.2497, -130)
  arc A123 through (38.1997, 125.85, -130) (38.3018, 127.0977, -130) (38.3634, 128.3481, -130)
  line L111 (32.4566, 147.6644, -130) -> (33.8365, 147.7851, -130)
  line L112 (35.7135, 120.3569, -130) -> (35.5372, 119.6991, -130)
  line L113 (28.9872, 106.3818, -130) -> (29.6268, 105.1532, -130)
  arc A124 through (-8.9153, 92.0699, -130) (-7.6916, 91.8058, -130) (-6.4599, 91.5815, -130)
  line L114 (36.6996, 124.0736, -130) -> (37.8678, 123.3294, -130)
  arc A125 through (-32.9053, 109.2517, -130) (-32.2267, 108.1997, -130) (-31.5144, 107.1702, -130)
  line L115 (34.5329, 115.9872, -130) -> (35.9167, 116.0476, -130)
  arc A126 through (6.1199, 91.5815, -130) (7.3516, 91.8058, -130) (8.5753, 92.0699, -130)
  line L116 (36.6155, 125.1198, -130) -> (36.5266, 124.4447, -130)
  line L117 (13.4621, 94.9164, -130) -> (13.4017, 93.5326, -130)
  line L118 (35.6603, 119.3086, -130) -> (36.7214, 118.4183, -130)
  line L119 (19.063, 97.6785, -130) -> (20.1976, 96.884, -130)
  line L120 (10.1407, 93.789, -130) -> (11.0311, 92.7279, -130)
  line L121 (23.0675, 100.4621, -130) -> (24.2961, 99.8226, -130)
  line L122 (37.1081, 130.3051, -130) -> (38.3634, 130.8905, -130)
  line L123 (32.0935, 111.3852, -130) -> (31.753, 110.7954, -130)
  line L124 (34.008, 114.72, -130) -> (34.9438, 113.6988, -130)
  arc A127 through (15.7505, 94.5056, -130) (16.8822, 95.041, -130) (17.9958, 95.6128, -130)
  arc A128 through (19.063, 97.6785, -130) (18.861, 97.747, -130) (18.6539, 97.6963, -130)
  line L125 (26.6745, 103.7447, -130) -> (27.9761, 103.2709, -130)
  line L126 (8.8159, 93.434, -130) -> (8.5753, 92.0699, -130)
  line L127 (31.7708, 110.3864, -130) -> (32.5653, 109.2517, -130)
  arc A129 through (13.6969, 95.2518, -130) (13.5306, 95.1184, -130) (13.4621, 94.9164, -130)
  arc A130 through (18.0642, 97.3558, -130) (17.9167, 97.2018, -130) (17.8751, 96.9927, -130)
  line L128 (29.4374, 107.3299, -130) -> (29.0229, 106.7897, -130)
  arc A131 through (31.1744, 107.1702, -130) (31.8868, 108.1997, -130) (32.5653, 109.2517, -130)
  arc A132 through (29.0229, 106.7897, -130) (28.9456, 106.5909, -130) (28.9872, 106.3818, -130)
  arc A133 through (22.1194, 100.0119, -130) (21.9933, 99.8399, -130) (21.9794, 99.6272, -130)
  arc A134 through (11.0311, 92.7279, -130) (12.2229, 93.111, -130) (13.4017, 93.5326, -130)
  line L129 (25.7046, 102.7748, -130) -> (26.1784, 101.4732, -130)
  line L130 (5.0046, 92.9227, -130) -> (4.3295, 92.8338, -130)
  line L131 (17.8751, 96.9927, -130) -> (17.9958, 95.6128, -130)
  line L132 (-22.3193, 99.6272, -130) -> (-22.6191, 98.2749, -130)
  line L133 (-26.1332, 103.1745, -130) -> (-26.6147, 103.6561, -130)
  arc A135 through (37.1081, 130.3051, -130) (36.9477, 130.1645, -130) (36.8881, 129.9598, -130)
  arc A136 through (34.5329, 115.9872, -130) (34.331, 115.9187, -130) (34.1975, 115.7524, -130)
  line L134 (31.7708, 148.8522, -130) -> (32.5653, 149.9869, -130)
  arc A137 through (36.8786, 125.4335, -130) (36.7014, 125.315, -130) (36.6155, 125.1198, -130)
  arc A138 through (-26.6147, 103.6561, -130) (-26.8017, 103.7586, -130) (-27.0145, 103.7447, -130)
  arc A139 through (-22.6191, 98.2749, -130) (-21.5896, 97.5625, -130) (-20.5375, 96.884, -130)
  arc A140 through (-13.7417, 93.5326, -130) (-12.5629, 93.111, -130) (-11.371, 92.7279, -130)
  line L135 (-29.3628, 106.7897, -130) -> (-29.7774, 107.3299, -130)
  arc A141 through (31.753, 110.7954, -130) (31.7023, 110.5883, -130) (31.7708, 110.3864, -130)
  line L136 (-13.8021, 94.9164, -130) -> (-13.7417, 93.5326, -130)
  arc A142 through (27.9761, 103.2709, -130) (28.8167, 104.1987, -130) (29.6268, 105.1532, -130)
  arc A143 through (38.3634, 130.8905, -130) (38.3018, 132.1409, -130) (38.1997, 133.3886, -130)
  arc A144 through (-13.8021, 94.9164, -130) (-13.8706, 95.1184, -130) (-14.0369, 95.2518, -130)
  line L137 (-27.0145, 103.7447, -130) -> (-28.3161, 103.2709, -130)
  line L138 (-19.4029, 97.6785, -130) -> (-20.5375, 96.884, -130)
  line L139 (-22.4594, 100.0119, -130) -> (-22.9996, 100.4265, -130)
  arc A145 through (35.9167, 116.0476, -130) (36.3383, 117.2264, -130) (36.7214, 118.4183, -130)
  arc A146 through (24.2961, 99.8226, -130) (25.2507, 100.6326, -130) (26.1784, 101.4732, -130)
  line L140 (26.2748, 103.6561, -130) -> (25.7932, 103.1745, -130)
  line L141 (32.4566, 111.5742, -130) -> (33.8365, 111.4535, -130)
  arc A147 through (-29.7774, 107.3299, -130) (-29.9493, 107.456, -130) (-30.1621, 107.47, -130)
  arc A148 through (36.8881, 129.2788, -130) (36.9477, 129.0741, -130) (37.1081, 128.9335, -130)
  arc A149 through (36.5266, 124.4447, -130) (36.559, 124.2339, -130) (36.6996, 124.0736, -130)
  line L142 (-14.0369, 95.2518, -130) -> (-14.6661, 95.5124, -130)
  line L143 (-23.4075, 100.4621, -130) -> (-24.6361, 99.8226, -130)
extrude "Extrude1''''" add sketch "Sketch1 (4)" along normal blind 10 separate body contours L0 L1 A0 L2 A1 A2 L3 L4 L5 L6 L7 L8 A3 A4 L9 L10 L11 L12 L13 A5 A6 A7 A8 A9 A10 A11 L14 L15 A12 A13 A14 A15 L16 L17 L18 L19 A17 L20 L21 L22 L23 L24 A18 A19 A20 A21 A22 A23 L25 L26 A24 A25 A26 L27 L28 L29 L30 L31 A27 A28 A29 A30 A31 A32 L32 L33 L34 A33 L35 L36 L37 A34 L38 A35 L39 A36 A37 L40 L41 A38 A39 A40 A41 L42 A42 L43 L44 L45 A43 A44 L46 L47 L48 A45 A46 A47 A48 L49 L50 L51 L52 A49 A50 L53 A51 L54 A52 L55 L56 A53 A54 L57 A55 A56 A57 A58 A59 A60 L58 L59 A61 A62 A63 A64 A65 A66 A67 A68 L60 L61 L62 A69 A70 A71 A72 L63 L64 L65 L66 L67 A73 A74 A79 A80 A81 L68 L69 L70 L71 A82 L72 L73 L74 A83 L75 L76 L77 A84 A85 A86 A87 A88 A89 L78 L79 A90 A91 L80 L81 L82 A92 A93 L83 A94 A95 L84 L85 L86 A96 L87 A97 L88 L89 A98 A99 L90 A100 A101 A102 A103 L91 L92 L93 L94 L95 L96 L97 L98 A104 L99 L100 A105 A106 A107 L101 L102 L103 L104 A108 A109 A110 L105 A111 A113 L106 A114 A115 L107 L108 L109 A116 A117 A118 L110 A119 A120 A121 A122 A123 L111 L112 L113 A124 L114 A125 L115 A126 L116 L117 L118 L119 L120 L121 L122 L123 L124 A127 A128 L125 L126 L127 A129 A130 L128 A131 A132 A133 A134 L129 L130 L131 L132 L133 A135 A136 L134 A137 A138 A139 A140 L135 A141 L136 A142 A143 A144 L137 L138 L139 A145 A146 L140 L141 A147 A148 A149 L142 L143 in plane through (-130, 0, 0) normal (1, 0, 0) makes body 5 in component "Large gear"
sketch "Sketch1 (5)" plane through (0, 0, 0) normal (0, 0, 1) x (1, 0, 0) in component "tilt tray"
  line L0 (-123, 30) -> (132, 30)
  line L1 (132, 30) -> (132, -30)
  line L2 (132, -30) -> (-123, -30)
  line L3 (-123, -30) -> (-123, 30)
  line L4 (132, 7.5) -> (138, 7.5)
  line L5 (138, 7.5) -> (138, 22.5)
  line L6 (138, 22.5) -> (132, 22.5)
  line L7 (132, 22.5) -> (132, 7.5)
  line L8 (138, -7.5) -> (132, -7.5)
  line L9 (138, -22.5) -> (138, -7.5)
  line L10 (132, -7.5) -> (132, -22.5)
  line L11 (132, -22.5) -> (138, -22.5)
  line L12 (-123, 22.5) -> (-129, 22.5)
  line L13 (-123, 7.5) -> (-123, 22.5)
  line L14 (-129, 22.5) -> (-129, 7.5)
  line L15 (-129, 7.5) -> (-123, 7.5)
  line L16 (-123, -7.5) -> (-129, -7.5)
  line L17 (-123, -22.5) -> (-123, -7.5)
  line L18 (-129, -7.5) -> (-129, -22.5)
  line L19 (-129, -22.5) -> (-123, -22.5)
  constraint horizontal L0
  constraint vertical L1
  constraint horizontal L2
  constraint vertical L3
  constraint horizontal L4
  constraint vertical L5
  constraint horizontal L6
  constraint vertical L7
  constraint horizontal L11
  constraint vertical L9
  constraint horizontal L8
  constraint vertical L10
  constraint horizontal L15
  constraint vertical L13
  constraint horizontal L12
  constraint vertical L14
  constraint horizontal L19
  constraint vertical L17
  constraint horizontal L16
  constraint vertical L18
extrude "Extrude1'''''" add sketch "Sketch1 (5)" along normal blind 6 separate body makes body 6 in component "tilt tray"
component "Base Tray" placed x (1, 0, 0) y (0, 1, 0) z (0, 0, 1) at (0, 0, 0)
component "Flange 2" placed x (1, 0, 0) y (0, 1, 0) z (0, 0, 1) at (0, 0, 0)
component "Flange 2" placed x (1, 0, 0) y (0, 1, 0) z (0, 0, 1) at (288, 0, 0)
component "Back support" placed x (1, 0, 0) y (0, 1, 0) z (0, 0, 1) at (0, 2, 0)
component "Tilt Flange 2" placed x (1, 0, 0) y (0, 1, 0) z (0, 0, 1) at (9, 0, 0)
component "Large gear" placed x (1, 0, 0) y (0, 1, 0) z (0, 0, 1) at (-10, 0, 0)
component "Tilt Flange 2" placed x (1, 0, 0) y (0, 1, 0) z (0, 0, 1) at (273, 0, 0)
component "tilt tray" placed x (1, 0, 0) y (0, 1, 0) z (0, 0, 1) at (0, 0, 57)
